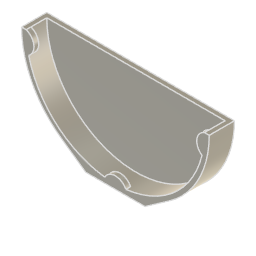
Improved Challenge Coin Holder (Autodesk Fusion 360 design; units mm, degrees)
Autodesk Fusion 360 part; units mm, degrees
sketch "Sketch1" plane through (0, 0, 0) normal (0, 0, 1) x (1, 0, 0)
  arc A0 (-23.75, 0) -> (23.75, 0) centre (0, 0) ccw
  line L0 (0, 0) -> (0, -23.75) construction
  line L1 (0, -23.75) -> (13.6224, -23.75)
  line L2 (0, -23.75) -> (-13.6224, -23.75)
  line L3 (23.75, 0) -> (22.55, 0)
  arc A1 (-22.55, 0) -> (22.55, 0) centre (0, 0) ccw
  line L4 (-23.75, 0) -> (-22.55, 0)
  line L5 (22.55, 0) -> (-22.55, 0)
  line L6 (-13.6224, -19.4549) -> (-25.9344, -10.8339) construction
  line L7 (-13.6224, -19.4549) -> (-13.6224, -23.75)
  line L8 (-13.6224, -19.4549) -> (-13.6224, -29.3622) construction
  line L9 (13.6224, -19.4549) -> (13.6224, -23.75)
  arc A2 (-23.0391, -5.7672) -> (-22.55, 0) centre (-23.5824, -2.8168) ccw
  arc A3 (3, -23.75) -> (-3, -23.75) centre (0, -23.75) ccw
  arc A4 (22.55, 0) -> (23.0391, -5.7672) centre (23.5824, -2.8168) ccw
  dimension "d1" = -1.2
  dimension "d2" = 55
  dimension "d3" = 3
  dimension "d4" = 22.55
  constraint coincident A0.centre L0.start
  constraint midpoint A0 L0.end
  constraint vertical L0
  constraint tangent A0 L1
  constraint perpendicular L0 L1
  constraint symmetric L1.start L0 L2.start
  constraint symmetric L0 L1.end L2.end
  constraint horizontal L3
  constraint symmetric A0.end L0 A0.start
  constraint symmetric L0 L3.end A1.start
  constraint parallel L4 L5
  constraint coincident A0 L6.start
  constraint tangent A0 L6
  constraint vertical L7
  constraint parallel L7 L8
  constraint coincident L2.end L7.end
  constraint symmetric L0 L6.start L9.start
  constraint symmetric L0 L2.end L1.end
  constraint coincident A0 A2.start
  constraint coincident A0 A2.centre
  constraint coincident L1 A3.start
  constraint coincident L2 A3.end
  constraint coincident L0.end L1.start
  constraint symmetric L0 A1.start L3.end
  constraint symmetric L0 A2.start A4.end
  constraint symmetric L0 A2 A4
  constraint midpoint A0.centre L5
  constraint equal A2 A3
  measures "d2" angle of L6 L8
  measures "d3" radius of A2
  measures "d4" radius of A1
extrude "Extrude1" add sketch "Sketch1" along normal blind 1.2
extrude "Extrude2" add sketch "Sketch1" along normal blind 4 from surface at 1.2 contours A0 A1 L4 A2 | A0 A1 A2 A3 | A0 L2 L7 A3 | A0 L3 A1 A4 | A0 A1 A3 | A0 L2 A3 | A0 A1 A3 A4 | A0 L1 A3 | A0 L1 L9 A3
extrude "Extrude3" add sketch "Sketch1" along normal blind 1.2 from surface at 5.2 contours A0 A1 L4 A2 | A0 A1 A2 A3 | A1 A2 | A0 L2 L7 A3 | A0 L3 A1 A4 | A1 A4 | A0 A1 A3 | A0 L2 A3 | A1 A3 | A0 A1 A3 A4 | A0 L1 A3 | A0 L1 L9 A3
sketch "Sketch2" plane through (0, 0, 6.4) normal (0, 0, 1) x (-1, 0, 0)
  line L0 (-13.6224, 23.75) -> (-13.6224, 19.4549)
  arc A0 (-13.6224, 19.4549) -> (-23.75, 0) centre (0, 0) ccw
  line L1 (-23.75, 0) -> (-22.55, 0)
  arc A1 (-22.55, 0) -> (-21.9156, 5.3112) centre (-23.5824, 2.8168) ccw
  arc A2 (-2.6745, 22.3908) -> (-21.9156, 5.3112) centre (0, 0) ccw
  arc A3 (-2.6745, 22.3908) -> (2.6745, 22.3908) centre (0, 23.75) ccw
  arc A4 (21.9156, 5.3112) -> (2.6745, 22.3908) centre (0, 0) ccw
  arc A5 (21.9156, 5.3112) -> (22.55, 0) centre (23.5824, 2.8168) ccw
  line L2 (22.55, 0) -> (23.75, 0)
  arc A6 (23.75, 0) -> (13.6224, 19.4549) centre (0, 0) ccw
  line L3 (13.6224, 19.4549) -> (13.6224, 23.75)
  line L4 (13.6224, 23.75) -> (-13.6224, 23.75)
  arc A7 (23.75, 0) -> (13.6224, 19.4549) centre (0, 0) ccw
  line L5 (13.6224, 23.75) -> (-13.6224, 23.75)
  line L6 (0, 23.75) -> (0, 21.8144) construction
  line L7 (13.6224, 19.4549) -> (7.4884, 23.75)
  line L8 (-13.6224, 19.4549) -> (-7.4884, 23.75)
  constraint coincident A3.centre L6.start
  constraint perpendicular L5 L6
  constraint coincident A6.end A7
  constraint coincident A6.end L3.start
  constraint tangent A7 L7
  constraint coincident L4 L7.end
  constraint symmetric L6 L7.end L8.end
  constraint symmetric L6 A6.end L0.end
extrude "Extrude4" cut sketch "Sketch2" against normal up to surface (6.4 mm away) contours L0 L4 L5 L8 | L3 L4 L5 L7
move_body "Move1" bodies 1 to x (1, 0, 0) y (0, 0, 1) z (0, -1, 0) at (0, -20.55, 26.95)
equation "d4 = ( 45.1 / 2 ) * 1 mm"
named bodies: "Improved Challenge Coin Holder"
